Autodesk Inventor part; units mm, degrees
(part 4 of 4)
sketch "Sketch7" plane through (0, 0, 2) normal (0, 0, 1) x (1, 0, 0)
  arc A0 (20.5, -320) -> (16, -320) centre (18.25, -320) ccw projected
  line L0 (20.5, -320) -> (20.5, -360) projected
  arc A1 (16, -360) -> (20.5, -360) centre (18.25, -360) ccw projected
  line L1 (16, -360) -> (16, -320) projected
  arc A2 (12.5, -320) -> (8, -320) centre (10.25, -320) ccw projected
  line L2 (12.5, -320) -> (12.5, -360) projected
  arc A3 (8, -360) -> (12.5, -360) centre (10.25, -360) ccw projected
  line L3 (8, -360) -> (8, -320) projected
  arc A4 (0, -360) -> (4.5, -360) centre (2.25, -360) ccw projected
  line L4 (0, -360) -> (0, -320) projected
  arc A5 (4.5, -320) -> (0, -320) centre (2.25, -320) ccw projected
  line L5 (4.5, -320) -> (4.5, -360) projected
  line L6 (283.7872, -294.4284) -> (283.7872, -329.9768) projected
  line L7 (283.7872, -329.9768) -> (273.4247, -329.9768) projected
  line L8 (273.4247, -329.9768) -> (267.105, -323.7035) projected
  line L9 (267.105, -323.7035) -> (267.105, -286.25) projected
  line L10 (267.105, -286.25) -> (273.4247, -279.9768) projected
  line L11 (273.4247, -279.9768) -> (299.54, -279.9768) projected
  line L12 (299.54, -279.9768) -> (299.54, -294.4284) projected
  line L13 (299.54, -294.4284) -> (283.7872, -294.4284) projected
  line L14 (242.9879, -315.1998) -> (242.9879, -330.0232) projected
  line L15 (242.9879, -330.0232) -> (227.2351, -330.0232) projected
  line L16 (227.2351, -330.0232) -> (210.553, -313.3411) projected
  line L17 (210.553, -313.3411) -> (210.553, -279.9768) projected
  line L18 (210.553, -279.9768) -> (227.2351, -279.9768) projected
  line L19 (227.2351, -279.9768) -> (227.2351, -315.1998) projected
  line L20 (227.2351, -315.1998) -> (242.9879, -315.1998) projected
  line L21 (206.2779, -316.1756) -> (206.2779, -329.9768) projected
  line L22 (206.2779, -329.9768) -> (173.8429, -329.9768) projected
  line L23 (173.8429, -329.9768) -> (173.8429, -316.1756) projected
  line L24 (173.8429, -316.1756) -> (206.2779, -316.1756) projected
  line L25 (170.3113, -279.9768) -> (170.3113, -329.9768) projected
  line L26 (170.3113, -329.9768) -> (159.9954, -329.9768) projected
  line L27 (159.9954, -329.9768) -> (153.7221, -323.7035) projected
  line L28 (153.7221, -323.7035) -> (153.7221, -286.25) projected
  line L29 (153.7221, -286.25) -> (159.9954, -279.9768) projected
  line L30 (159.9954, -279.9768) -> (170.3113, -279.9768) projected
  line L31 (129.3262, -316.1292) -> (129.3262, -329.9303) projected
  line L32 (129.3262, -329.9303) -> (104.7444, -329.9303) projected
  line L33 (104.7444, -329.9303) -> (96.8913, -322.0771) projected
  line L34 (96.8913, -322.0771) -> (96.8913, -294.289) projected
  line L35 (96.8913, -294.289) -> (113.5734, -294.289) projected
  line L36 (113.5734, -294.289) -> (113.5734, -316.1292) projected
  line L37 (113.5734, -316.1292) -> (129.3262, -316.1292) projected
  line L38 (56.789, -329.9768) -> (46.6125, -329.9768) projected
  line L39 (46.6125, -329.9768) -> (40.3392, -323.7035) projected
  line L40 (40.3392, -323.7035) -> (40.3392, -279.9768) projected
  line L41 (40.3392, -279.9768) -> (56.789, -279.9768) projected
  line L42 (56.789, -279.9768) -> (56.789, -329.9768) projected
  line L43 (92.5697, -329.9768) -> (60.3206, -329.9768) projected
  line L44 (60.3206, -329.9768) -> (60.3206, -316.1756) projected
  line L45 (60.3206, -316.1756) -> (92.5697, -316.1756) projected
  line L46 (92.5697, -316.1756) -> (92.5697, -329.9768) projected
  line L47 (149.447, -294.289) -> (149.447, -329.9303) projected
  line L48 (149.447, -329.9303) -> (132.7649, -329.9303) projected
  line L49 (132.7649, -329.9303) -> (132.7649, -294.289) projected
  line L50 (132.7649, -294.289) -> (149.447, -294.289) projected
  line L51 (206.2779, -279.9768) -> (206.2779, -294.4284) projected
  line L52 (206.2779, -294.4284) -> (173.8429, -294.4284) projected
  line L53 (173.8429, -294.4284) -> (173.8429, -279.9768) projected
  line L54 (173.8429, -279.9768) -> (206.2779, -279.9768) projected
  line L55 (206.2779, -297.96) -> (206.2779, -308.973) projected
  line L56 (206.2779, -308.973) -> (173.8429, -308.973) projected
  line L57 (173.8429, -308.973) -> (173.8429, -297.96) projected
  line L58 (173.8429, -297.96) -> (206.2779, -297.96) projected
  line L59 (262.8299, -313.3411) -> (246.4266, -329.9768) projected
  line L60 (246.4266, -329.9768) -> (246.4266, -279.9768) projected
  line L61 (246.4266, -279.9768) -> (262.8299, -279.9768) projected
  line L62 (262.8299, -279.9768) -> (262.8299, -313.3411) projected
  line L63 (319.6608, -286.25) -> (319.6608, -323.7035) projected
  line L64 (319.6608, -323.7035) -> (313.3411, -329.9768) projected
  line L65 (313.3411, -329.9768) -> (287.1794, -329.9768) projected
  line L66 (287.1794, -329.9768) -> (287.1794, -316.1756) projected
  line L67 (287.1794, -316.1756) -> (302.9786, -316.1756) projected
  line L68 (302.9786, -316.1756) -> (302.9786, -279.9768) projected
  line L69 (302.9786, -279.9768) -> (313.3411, -279.9768) projected
  line L70 (313.3411, -279.9768) -> (319.6608, -286.25) projected
  line L71 (31.2247, -413) -> (28.338, -408) projected
  line L72 (28.338, -408) -> (31.2247, -403) projected
  line L73 (31.2247, -403) -> (36.9983, -403) projected
  line L74 (36.9983, -403) -> (39.885, -408) projected
  line L75 (39.885, -408) -> (36.9983, -413) projected
  line L76 (36.9983, -413) -> (31.2247, -413) projected
  line L77 (49.9886, -440.5) -> (52.8754, -445.5) projected
  line L78 (52.8754, -445.5) -> (49.9886, -450.5) projected
  line L79 (49.9886, -450.5) -> (44.2151, -450.5) projected
  line L80 (44.2151, -450.5) -> (41.3284, -445.5) projected
  line L81 (41.3284, -445.5) -> (44.2151, -440.5) projected
  line L82 (44.2151, -440.5) -> (49.9886, -440.5) projected
  line L83 (57.2247, -418) -> (62.9983, -418) projected
  line L84 (62.9983, -418) -> (65.885, -423) projected
  line L85 (65.885, -423) -> (62.9983, -428) projected
  line L86 (62.9983, -428) -> (57.2247, -428) projected
  line L87 (57.2247, -428) -> (54.338, -423) projected
  line L88 (54.338, -423) -> (57.2247, -418) projected
  line L89 (78.8754, -430.5) -> (75.9886, -435.5) projected
  line L90 (75.9886, -435.5) -> (70.2151, -435.5) projected
  line L91 (70.2151, -435.5) -> (67.3284, -430.5) projected
  line L92 (67.3284, -430.5) -> (70.2151, -425.5) projected
  line L93 (70.2151, -425.5) -> (75.9886, -425.5) projected
  line L94 (75.9886, -425.5) -> (78.8754, -430.5) projected
  line L95 (80.338, -438) -> (83.2247, -433) projected
  line L96 (83.2247, -433) -> (88.9983, -433) projected
  line L97 (88.9983, -433) -> (91.885, -438) projected
  line L98 (91.885, -438) -> (88.9983, -443) projected
  line L99 (88.9983, -443) -> (83.2247, -443) projected
  line L100 (83.2247, -443) -> (80.338, -438) projected
  line L101 (101.9886, -410.5) -> (104.8754, -415.5) projected
  line L102 (104.8754, -415.5) -> (101.9886, -420.5) projected
  line L103 (101.9886, -420.5) -> (96.2151, -420.5) projected
  line L104 (96.2151, -420.5) -> (93.3284, -415.5) projected
  line L105 (93.3284, -415.5) -> (96.2151, -410.5) projected
  line L106 (96.2151, -410.5) -> (101.9886, -410.5) projected
  line L107 (109.2247, -448) -> (114.9983, -448) projected
  line L108 (114.9983, -448) -> (117.885, -453) projected
  line L109 (117.885, -453) -> (114.9983, -458) projected
  line L110 (114.9983, -458) -> (109.2247, -458) projected
  line L111 (109.2247, -458) -> (106.338, -453) projected
  line L112 (106.338, -453) -> (109.2247, -448) projected
  line L113 (135.2247, -413) -> (132.338, -408) projected
  line L114 (132.338, -408) -> (135.2247, -403) projected
  line L115 (135.2247, -403) -> (140.9983, -403) projected
  line L116 (140.9983, -403) -> (143.885, -408) projected
  line L117 (143.885, -408) -> (140.9983, -413) projected
  line L118 (140.9983, -413) -> (135.2247, -413) projected
  line L119 (153.9886, -440.5) -> (156.8754, -445.5) projected
  line L120 (156.8754, -445.5) -> (153.9886, -450.5) projected
  line L121 (153.9886, -450.5) -> (148.2151, -450.5) projected
  line L122 (148.2151, -450.5) -> (145.3284, -445.5) projected
  line L123 (145.3284, -445.5) -> (148.2151, -440.5) projected
  line L124 (148.2151, -440.5) -> (153.9886, -440.5) projected
  line L125 (153.9886, -410.5) -> (156.8754, -415.5) projected
  line L126 (156.8754, -415.5) -> (153.9886, -420.5) projected
  line L127 (153.9886, -420.5) -> (148.2151, -420.5) projected
  line L128 (148.2151, -420.5) -> (145.3284, -415.5) projected
  line L129 (145.3284, -415.5) -> (148.2151, -410.5) projected
  line L130 (148.2151, -410.5) -> (153.9886, -410.5) projected
  line L131 (182.8754, -430.5) -> (179.9886, -435.5) projected
  line L132 (179.9886, -435.5) -> (174.2151, -435.5) projected
  line L133 (174.2151, -435.5) -> (171.3284, -430.5) projected
  line L134 (171.3284, -430.5) -> (174.2151, -425.5) projected
  line L135 (174.2151, -425.5) -> (179.9886, -425.5) projected
  line L136 (179.9886, -425.5) -> (182.8754, -430.5) projected
  line L137 (184.338, -438) -> (187.2247, -433) projected
  line L138 (187.2247, -433) -> (192.9983, -433) projected
  line L139 (192.9983, -433) -> (195.885, -438) projected
  line L140 (195.885, -438) -> (192.9983, -443) projected
  line L141 (192.9983, -443) -> (187.2247, -443) projected
  line L142 (187.2247, -443) -> (184.338, -438) projected
  line L143 (205.9886, -410.5) -> (208.8754, -415.5) projected
  line L144 (208.8754, -415.5) -> (205.9886, -420.5) projected
  line L145 (205.9886, -420.5) -> (200.2151, -420.5) projected
  line L146 (200.2151, -420.5) -> (197.3284, -415.5) projected
  line L147 (197.3284, -415.5) -> (200.2151, -410.5) projected
  line L148 (200.2151, -410.5) -> (205.9886, -410.5) projected
  line L149 (213.2247, -448) -> (218.9983, -448) projected
  line L150 (218.9983, -448) -> (221.885, -453) projected
  line L151 (221.885, -453) -> (218.9983, -458) projected
  line L152 (218.9983, -458) -> (213.2247, -458) projected
  line L153 (213.2247, -458) -> (210.338, -453) projected
  line L154 (210.338, -453) -> (213.2247, -448) projected
  line L155 (239.2247, -413) -> (236.338, -408) projected
  line L156 (236.338, -408) -> (239.2247, -403) projected
  line L157 (239.2247, -403) -> (244.9983, -403) projected
  line L158 (244.9983, -403) -> (247.885, -408) projected
  line L159 (247.885, -408) -> (244.9983, -413) projected
  line L160 (244.9983, -413) -> (239.2247, -413) projected
  line L161 (257.9886, -440.5) -> (260.8754, -445.5) projected
  line L162 (260.8754, -445.5) -> (257.9886, -450.5) projected
  line L163 (257.9886, -450.5) -> (252.2151, -450.5) projected
  line L164 (252.2151, -450.5) -> (249.3284, -445.5) projected
  line L165 (249.3284, -445.5) -> (252.2151, -440.5) projected
  line L166 (252.2151, -440.5) -> (257.9886, -440.5) projected
  line L167 (265.2247, -418) -> (270.9983, -418) projected
  line L168 (270.9983, -418) -> (273.885, -423) projected
  line L169 (273.885, -423) -> (270.9983, -428) projected
  line L170 (270.9983, -428) -> (265.2247, -428) projected
  line L171 (265.2247, -428) -> (262.338, -423) projected
  line L172 (262.338, -423) -> (265.2247, -418) projected
  line L173 (291.2247, -448) -> (296.9983, -448) projected
  line L174 (296.9983, -448) -> (299.885, -453) projected
  line L175 (299.885, -453) -> (296.9983, -458) projected
  line L176 (296.9983, -458) -> (291.2247, -458) projected
  line L177 (291.2247, -458) -> (288.338, -453) projected
  line L178 (288.338, -453) -> (291.2247, -448) projected
  line L179 (343.2247, -448) -> (348.9983, -448) projected
  line L180 (348.9983, -448) -> (351.885, -453) projected
  line L181 (351.885, -453) -> (348.9983, -458) projected
  line L182 (348.9983, -458) -> (343.2247, -458) projected
  line L183 (343.2247, -458) -> (340.338, -453) projected
  line L184 (340.338, -453) -> (343.2247, -448) projected
  line L185 (335.9886, -410.5) -> (338.8754, -415.5) projected
  line L186 (338.8754, -415.5) -> (335.9886, -420.5) projected
  line L187 (335.9886, -420.5) -> (330.2151, -420.5) projected
  line L188 (330.2151, -420.5) -> (327.3284, -415.5) projected
  line L189 (327.3284, -415.5) -> (330.2151, -410.5) projected
  line L190 (330.2151, -410.5) -> (335.9886, -410.5) projected
  line L191 (286.8754, -430.5) -> (283.9886, -435.5) projected
  line L192 (283.9886, -435.5) -> (278.2151, -435.5) projected
  line L193 (278.2151, -435.5) -> (275.3284, -430.5) projected
  line L194 (275.3284, -430.5) -> (278.2151, -425.5) projected
  line L195 (278.2151, -425.5) -> (283.9886, -425.5) projected
  line L196 (283.9886, -425.5) -> (286.8754, -430.5) projected
  line L197 (309.9886, -410.5) -> (312.8754, -415.5) projected
  line L198 (312.8754, -415.5) -> (309.9886, -420.5) projected
  line L199 (309.9886, -420.5) -> (304.2151, -420.5) projected
  line L200 (304.2151, -420.5) -> (301.3284, -415.5) projected
  line L201 (301.3284, -415.5) -> (304.2151, -410.5) projected
  line L202 (304.2151, -410.5) -> (309.9886, -410.5) projected
  line L203 (5.2247, -433) -> (10.9983, -433) projected
  line L204 (10.9983, -433) -> (13.885, -438) projected
  line L205 (13.885, -438) -> (10.9983, -443) projected
  line L206 (10.9983, -443) -> (5.2247, -443) projected
  line L207 (5.2247, -443) -> (2.338, -438) projected
  line L208 (2.338, -438) -> (5.2247, -433) projected
  line L209 (23.9886, -440.5) -> (26.8754, -445.5) projected
  line L210 (26.8754, -445.5) -> (23.9886, -450.5) projected
  line L211 (23.9886, -450.5) -> (18.2151, -450.5) projected
  line L212 (18.2151, -450.5) -> (15.3284, -445.5) projected
  line L213 (15.3284, -445.5) -> (18.2151, -440.5) projected
  line L214 (18.2151, -440.5) -> (23.9886, -440.5) projected
  line L215 (10.9983, -428) -> (5.2247, -428) projected
  line L216 (5.2247, -428) -> (2.338, -423) projected
  line L217 (2.338, -423) -> (5.2247, -418) projected
  line L218 (5.2247, -418) -> (10.9983, -418) projected
  line L219 (10.9983, -418) -> (13.885, -423) projected
  line L220 (13.885, -423) -> (10.9983, -428) projected
  line L221 (317.2247, -418) -> (322.9983, -418) projected
  line L222 (322.9983, -418) -> (325.885, -423) projected
  line L223 (325.885, -423) -> (322.9983, -428) projected
  line L224 (322.9983, -428) -> (317.2247, -428) projected
  line L225 (317.2247, -428) -> (314.338, -423) projected
  line L226 (314.338, -423) -> (317.2247, -418) projected
  line L227 (291.2247, -418) -> (296.9983, -418) projected
  line L228 (296.9983, -418) -> (299.885, -423) projected
  line L229 (299.885, -423) -> (296.9983, -428) projected
  line L230 (296.9983, -428) -> (291.2247, -428) projected
  line L231 (291.2247, -428) -> (288.338, -423) projected
  line L232 (288.338, -423) -> (291.2247, -418) projected
  line L233 (317.2247, -413) -> (314.338, -408) projected
  line L234 (314.338, -408) -> (317.2247, -403) projected
  line L235 (317.2247, -403) -> (322.9983, -403) projected
  line L236 (322.9983, -403) -> (325.885, -408) projected
  line L237 (325.885, -408) -> (322.9983, -413) projected
  line L238 (322.9983, -413) -> (317.2247, -413) projected
  line L239 (340.338, -438) -> (343.2247, -433) projected
  line L240 (343.2247, -433) -> (348.9983, -433) projected
  line L241 (348.9983, -433) -> (351.885, -438) projected
  line L242 (351.885, -438) -> (348.9983, -443) projected
  line L243 (348.9983, -443) -> (343.2247, -443) projected
  line L244 (343.2247, -443) -> (340.338, -438) projected
  line L245 (309.9886, -440.5) -> (312.8754, -445.5) projected
  line L246 (312.8754, -445.5) -> (309.9886, -450.5) projected
  line L247 (309.9886, -450.5) -> (304.2151, -450.5) projected
  line L248 (304.2151, -450.5) -> (301.3284, -445.5) projected
  line L249 (301.3284, -445.5) -> (304.2151, -440.5) projected
  line L250 (304.2151, -440.5) -> (309.9886, -440.5) projected
  line L251 (262.338, -438) -> (265.2247, -433) projected
  line L252 (265.2247, -433) -> (270.9983, -433) projected
  line L253 (270.9983, -433) -> (273.885, -438) projected
  line L254 (273.885, -438) -> (270.9983, -443) projected
  line L255 (270.9983, -443) -> (265.2247, -443) projected
  line L256 (265.2247, -443) -> (262.338, -438) projected
  line L257 (260.8754, -430.5) -> (257.9886, -435.5) projected
  line L258 (257.9886, -435.5) -> (252.2151, -435.5) projected
  line L259 (252.2151, -435.5) -> (249.3284, -430.5) projected
  line L260 (249.3284, -430.5) -> (252.2151, -425.5) projected
  line L261 (252.2151, -425.5) -> (257.9886, -425.5) projected
  line L262 (257.9886, -425.5) -> (260.8754, -430.5) projected
  line L263 (239.2247, -418) -> (244.9983, -418) projected
  line L264 (244.9983, -418) -> (247.885, -423) projected
  line L265 (247.885, -423) -> (244.9983, -428) projected
  line L266 (244.9983, -428) -> (239.2247, -428) projected
  line L267 (239.2247, -428) -> (236.338, -423) projected
  line L268 (236.338, -423) -> (239.2247, -418) projected
  line L269 (231.9886, -440.5) -> (234.8754, -445.5) projected
  line L270 (234.8754, -445.5) -> (231.9886, -450.5) projected
  line L271 (231.9886, -450.5) -> (226.2151, -450.5) projected
  line L272 (226.2151, -450.5) -> (223.3284, -445.5) projected
  line L273 (223.3284, -445.5) -> (226.2151, -440.5) projected
  line L274 (226.2151, -440.5) -> (231.9886, -440.5) projected
  line L275 (213.2247, -413) -> (210.338, -408) projected
  line L276 (210.338, -408) -> (213.2247, -403) projected
  line L277 (213.2247, -403) -> (218.9983, -403) projected
  line L278 (218.9983, -403) -> (221.885, -408) projected
  line L279 (221.885, -408) -> (218.9983, -413) projected
  line L280 (218.9983, -413) -> (213.2247, -413) projected
  line L281 (187.2247, -448) -> (192.9983, -448) projected
  line L282 (192.9983, -448) -> (195.885, -453) projected
  line L283 (195.885, -453) -> (192.9983, -458) projected
  line L284 (192.9983, -458) -> (187.2247, -458) projected
  line L285 (187.2247, -458) -> (184.338, -453) projected
  line L286 (184.338, -453) -> (187.2247, -448) projected
  line L287 (179.9886, -410.5) -> (182.8754, -415.5) projected
  line L288 (182.8754, -415.5) -> (179.9886, -420.5) projected
  line L289 (179.9886, -420.5) -> (174.2151, -420.5) projected
  line L290 (174.2151, -420.5) -> (171.3284, -415.5) projected
  line L291 (171.3284, -415.5) -> (174.2151, -410.5) projected
  line L292 (174.2151, -410.5) -> (179.9886, -410.5) projected
  line L293 (161.2247, -413) -> (158.338, -408) projected
  line L294 (158.338, -408) -> (161.2247, -403) projected
  line L295 (161.2247, -403) -> (166.9983, -403) projected
  line L296 (166.9983, -403) -> (169.885, -408) projected
  line L297 (169.885, -408) -> (166.9983, -413) projected
  line L298 (166.9983, -413) -> (161.2247, -413) projected
  line L299 (161.2247, -448) -> (166.9983, -448) projected
  line L300 (166.9983, -448) -> (169.885, -453) projected
  line L301 (169.885, -453) -> (166.9983, -458) projected
  line L302 (166.9983, -458) -> (161.2247, -458) projected
  line L303 (161.2247, -458) -> (158.338, -453) projected
  line L304 (158.338, -453) -> (161.2247, -448) projected
  line L305 (135.2247, -418) -> (140.9983, -418) projected
  line L306 (140.9983, -418) -> (143.885, -423) projected
  line L307 (143.885, -423) -> (140.9983, -428) projected
  line L308 (140.9983, -428) -> (135.2247, -428) projected
  line L309 (135.2247, -428) -> (132.338, -423) projected
  line L310 (132.338, -423) -> (135.2247, -418) projected
  line L311 (127.9886, -440.5) -> (130.8754, -445.5) projected
  line L312 (130.8754, -445.5) -> (127.9886, -450.5) projected
  line L313 (127.9886, -450.5) -> (122.2151, -450.5) projected
  line L314 (122.2151, -450.5) -> (119.3284, -445.5) projected
  line L315 (119.3284, -445.5) -> (122.2151, -440.5) projected
  line L316 (122.2151, -440.5) -> (127.9886, -440.5) projected
  line L317 (109.2247, -413) -> (106.338, -408) projected
  line L318 (106.338, -408) -> (109.2247, -403) projected
  line L319 (109.2247, -403) -> (114.9983, -403) projected
  line L320 (114.9983, -403) -> (117.885, -408) projected
  line L321 (117.885, -408) -> (114.9983, -413) projected
  line L322 (114.9983, -413) -> (109.2247, -413) projected
  line L323 (83.2247, -448) -> (88.9983, -448) projected
  line L324 (88.9983, -448) -> (91.885, -453) projected
  line L325 (91.885, -453) -> (88.9983, -458) projected
  line L326 (88.9983, -458) -> (83.2247, -458) projected
  line L327 (83.2247, -458) -> (80.338, -453) projected
  line L328 (80.338, -453) -> (83.2247, -448) projected
  line L329 (75.9886, -410.5) -> (78.8754, -415.5) projected
  line L330 (78.8754, -415.5) -> (75.9886, -420.5) projected
  line L331 (75.9886, -420.5) -> (70.2151, -420.5) projected
  line L332 (70.2151, -420.5) -> (67.3284, -415.5) projected
  line L333 (67.3284, -415.5) -> (70.2151, -410.5) projected
  line L334 (70.2151, -410.5) -> (75.9886, -410.5) projected
  line L335 (54.338, -438) -> (57.2247, -433) projected
  line L336 (57.2247, -433) -> (62.9983, -433) projected
  line L337 (62.9983, -433) -> (65.885, -438) projected
  line L338 (65.885, -438) -> (62.9983, -443) projected
  line L339 (62.9983, -443) -> (57.2247, -443) projected
  line L340 (57.2247, -443) -> (54.338, -438) projected
  line L341 (52.8754, -430.5) -> (49.9886, -435.5) projected
  line L342 (49.9886, -435.5) -> (44.2151, -435.5) projected
  line L343 (44.2151, -435.5) -> (41.3284, -430.5) projected
  line L344 (41.3284, -430.5) -> (44.2151, -425.5) projected
  line L345 (44.2151, -425.5) -> (49.9886, -425.5) projected
  line L346 (49.9886, -425.5) -> (52.8754, -430.5) projected
  line L347 (31.2247, -418) -> (36.9983, -418) projected
  line L348 (36.9983, -418) -> (39.885, -423) projected
  line L349 (39.885, -423) -> (36.9983, -428) projected
  line L350 (36.9983, -428) -> (31.2247, -428) projected
  line L351 (31.2247, -428) -> (28.338, -423) projected
  line L352 (28.338, -423) -> (31.2247, -418) projected
  line L353 (23.9886, -420.5) -> (18.2151, -420.5) projected
  line L354 (18.2151, -420.5) -> (15.3284, -415.5) projected
  line L355 (15.3284, -415.5) -> (18.2151, -410.5) projected
  line L356 (18.2151, -410.5) -> (23.9886, -410.5) projected
  line L357 (23.9886, -410.5) -> (26.8754, -415.5) projected
  line L358 (26.8754, -415.5) -> (23.9886, -420.5) projected
  line L359 (31.2247, -448) -> (36.9983, -448) projected
  line L360 (36.9983, -448) -> (39.885, -453) projected
  line L361 (39.885, -453) -> (36.9983, -458) projected
  line L362 (36.9983, -458) -> (31.2247, -458) projected
  line L363 (31.2247, -458) -> (28.338, -453) projected
  line L364 (28.338, -453) -> (31.2247, -448) projected
  line L365 (57.2247, -413) -> (54.338, -408) projected
  line L366 (54.338, -408) -> (57.2247, -403) projected
  line L367 (57.2247, -403) -> (62.9983, -403) projected
  line L368 (62.9983, -403) -> (65.885, -408) projected
  line L369 (65.885, -408) -> (62.9983, -413) projected
  line L370 (62.9983, -413) -> (57.2247, -413) projected
  line L371 (75.9886, -440.5) -> (78.8754, -445.5) projected
  line L372 (78.8754, -445.5) -> (75.9886, -450.5) projected
  line L373 (75.9886, -450.5) -> (70.2151, -450.5) projected
  line L374 (70.2151, -450.5) -> (67.3284, -445.5) projected
  line L375 (67.3284, -445.5) -> (70.2151, -440.5) projected
  line L376 (70.2151, -440.5) -> (75.9886, -440.5) projected
  line L377 (83.2247, -418) -> (88.9983, -418) projected
  line L378 (88.9983, -418) -> (91.885, -423) projected
  line L379 (91.885, -423) -> (88.9983, -428) projected
  line L380 (88.9983, -428) -> (83.2247, -428) projected
  line L381 (83.2247, -428) -> (80.338, -423) projected
  line L382 (80.338, -423) -> (83.2247, -418) projected
  line L383 (104.8754, -430.5) -> (101.9886, -435.5) projected
  line L384 (101.9886, -435.5) -> (96.2151, -435.5) projected
  line L385 (96.2151, -435.5) -> (93.3284, -430.5) projected
  line L386 (93.3284, -430.5) -> (96.2151, -425.5) projected
  line L387 (96.2151, -425.5) -> (101.9886, -425.5) projected
  line L388 (101.9886, -425.5) -> (104.8754, -430.5) projected
  line L389 (106.338, -438) -> (109.2247, -433) projected
  line L390 (109.2247, -433) -> (114.9983, -433) projected
  line L391 (114.9983, -433) -> (117.885, -438) projected
  line L392 (117.885, -438) -> (114.9983, -443) projected
  line L393 (114.9983, -443) -> (109.2247, -443) projected
  line L394 (109.2247, -443) -> (106.338, -438) projected
  line L395 (127.9886, -410.5) -> (130.8754, -415.5) projected
  line L396 (130.8754, -415.5) -> (127.9886, -420.5) projected
  line L397 (127.9886, -420.5) -> (122.2151, -420.5) projected
  line L398 (122.2151, -420.5) -> (119.3284, -415.5) projected
  line L399 (119.3284, -415.5) -> (122.2151, -410.5) projected
  line L400 (122.2151, -410.5) -> (127.9886, -410.5) projected
  line L401 (135.2247, -448) -> (140.9983, -448) projected
  line L402 (140.9983, -448) -> (143.885, -453) projected
  line L403 (143.885, -453) -> (140.9983, -458) projected
  line L404 (140.9983, -458) -> (135.2247, -458) projected
  line L405 (135.2247, -458) -> (132.338, -453) projected
  line L406 (132.338, -453) -> (135.2247, -448) projected
  line L407 (156.8754, -430.5) -> (153.9886, -435.5) projected
  line L408 (153.9886, -435.5) -> (148.2151, -435.5) projected
  line L409 (148.2151, -435.5) -> (145.3284, -430.5) projected
  line L410 (145.3284, -430.5) -> (148.2151, -425.5) projected
  line L411 (148.2151, -425.5) -> (153.9886, -425.5) projected
  line L412 (153.9886, -425.5) -> (156.8754, -430.5) projected
  line L413 (179.9886, -440.5) -> (182.8754, -445.5) projected
  line L414 (182.8754, -445.5) -> (179.9886, -450.5) projected
  line L415 (179.9886, -450.5) -> (174.2151, -450.5) projected
  line L416 (174.2151, -450.5) -> (171.3284, -445.5) projected
  line L417 (171.3284, -445.5) -> (174.2151, -440.5) projected
  line L418 (174.2151, -440.5) -> (179.9886, -440.5) projected
  line L419 (187.2247, -418) -> (192.9983, -418) projected
  line L420 (192.9983, -418) -> (195.885, -423) projected
  line L421 (195.885, -423) -> (192.9983, -428) projected
  line L422 (192.9983, -428) -> (187.2247, -428) projected
  line L423 (187.2247, -428) -> (184.338, -423) projected
  line L424 (184.338, -423) -> (187.2247, -418) projected
  line L425 (208.8754, -430.5) -> (205.9886, -435.5) projected
  line L426 (205.9886, -435.5) -> (200.2151, -435.5) projected
  line L427 (200.2151, -435.5) -> (197.3284, -430.5) projected
  line L428 (197.3284, -430.5) -> (200.2151, -425.5) projected
  line L429 (200.2151, -425.5) -> (205.9886, -425.5) projected
  line L430 (205.9886, -425.5) -> (208.8754, -430.5) projected
  line L431 (210.338, -438) -> (213.2247, -433) projected
  line L432 (213.2247, -433) -> (218.9983, -433) projected
  line L433 (218.9983, -433) -> (221.885, -438) projected
  line L434 (221.885, -438) -> (218.9983, -443) projected
  line L435 (218.9983, -443) -> (213.2247, -443) projected
  line L436 (213.2247, -443) -> (210.338, -438) projected
  line L437 (231.9886, -410.5) -> (234.8754, -415.5) projected
  line L438 (234.8754, -415.5) -> (231.9886, -420.5) projected
  line L439 (231.9886, -420.5) -> (226.2151, -420.5) projected
  line L440 (226.2151, -420.5) -> (223.3284, -415.5) projected
  line L441 (223.3284, -415.5) -> (226.2151, -410.5) projected
  line L442 (226.2151, -410.5) -> (231.9886, -410.5) projected
  line L443 (239.2247, -448) -> (244.9983, -448) projected
  line L444 (244.9983, -448) -> (247.885, -453) projected
  line L445 (247.885, -453) -> (244.9983, -458) projected
  line L446 (244.9983, -458) -> (239.2247, -458) projected
  line L447 (239.2247, -458) -> (236.338, -453) projected
  line L448 (236.338, -453) -> (239.2247, -448) projected
  line L449 (265.2247, -413) -> (262.338, -408) projected
  line L450 (262.338, -408) -> (265.2247, -403) projected
  line L451 (265.2247, -403) -> (270.9983, -403) projected
  line L452 (270.9983, -403) -> (273.885, -408) projected
  line L453 (273.885, -408) -> (270.9983, -413) projected
  line L454 (270.9983, -413) -> (265.2247, -413) projected
  line L455 (283.9886, -440.5) -> (286.8754, -445.5) projected
  line L456 (286.8754, -445.5) -> (283.9886, -450.5) projected
  line L457 (283.9886, -450.5) -> (278.2151, -450.5) projected
  line L458 (278.2151, -450.5) -> (275.3284, -445.5) projected
  line L459 (275.3284, -445.5) -> (278.2151, -440.5) projected
  line L460 (278.2151, -440.5) -> (283.9886, -440.5) projected
  line L461 (335.9886, -440.5) -> (338.8754, -445.5) projected
  line L462 (338.8754, -445.5) -> (335.9886, -450.5) projected
  line L463 (335.9886, -450.5) -> (330.2151, -450.5) projected
  line L464 (330.2151, -450.5) -> (327.3284, -445.5) projected
  line L465 (327.3284, -445.5) -> (330.2151, -440.5) projected
  line L466 (330.2151, -440.5) -> (335.9886, -440.5) projected
  line L467 (343.2247, -413) -> (340.338, -408) projected
  line L468 (340.338, -408) -> (343.2247, -403) projected
  line L469 (343.2247, -403) -> (348.9983, -403) projected
  line L470 (348.9983, -403) -> (351.885, -408) projected
  line L471 (351.885, -408) -> (348.9983, -413) projected
  line L472 (348.9983, -413) -> (343.2247, -413) projected
  line L473 (283.9886, -410.5) -> (286.8754, -415.5) projected
  line L474 (286.8754, -415.5) -> (283.9886, -420.5) projected
  line L475 (283.9886, -420.5) -> (278.2151, -420.5) projected
  line L476 (278.2151, -420.5) -> (275.3284, -415.5) projected
  line L477 (275.3284, -415.5) -> (278.2151, -410.5) projected
  line L478 (278.2151, -410.5) -> (283.9886, -410.5) projected
  line L479 (312.8754, -430.5) -> (309.9886, -435.5) projected
  line L480 (309.9886, -435.5) -> (304.2151, -435.5) projected
  line L481 (304.2151, -435.5) -> (301.3284, -430.5) projected
  line L482 (301.3284, -430.5) -> (304.2151, -425.5) projected
  line L483 (304.2151, -425.5) -> (309.9886, -425.5) projected
  line L484 (309.9886, -425.5) -> (312.8754, -430.5) projected
  line L485 (338.8754, -430.5) -> (335.9886, -435.5) projected
  line L486 (335.9886, -435.5) -> (330.2151, -435.5) projected
  line L487 (330.2151, -435.5) -> (327.3284, -430.5) projected
  line L488 (327.3284, -430.5) -> (330.2151, -425.5) projected
  line L489 (330.2151, -425.5) -> (335.9886, -425.5) projected
  line L490 (335.9886, -425.5) -> (338.8754, -430.5) projected
  line L491 (23.9886, -435.5) -> (18.2151, -435.5) projected
  line L492 (18.2151, -435.5) -> (15.3284, -430.5) projected
  line L493 (15.3284, -430.5) -> (18.2151, -425.5) projected
  line L494 (18.2151, -425.5) -> (23.9886, -425.5) projected
  line L495 (23.9886, -425.5) -> (26.8754, -430.5) projected
  line L496 (26.8754, -430.5) -> (23.9886, -435.5) projected
  line L497 (5.2247, -448) -> (10.9983, -448) projected
  line L498 (10.9983, -448) -> (13.885, -453) projected
  line L499 (13.885, -453) -> (10.9983, -458) projected
  line L500 (10.9983, -458) -> (5.2247, -458) projected
  line L501 (5.2247, -458) -> (2.338, -453) projected
  line L502 (2.338, -453) -> (5.2247, -448) projected
  line L503 (314.338, -438) -> (317.2247, -433) projected
  line L504 (317.2247, -433) -> (322.9983, -433) projected
  line L505 (322.9983, -433) -> (325.885, -438) projected
  line L506 (325.885, -438) -> (322.9983, -443) projected
  line L507 (322.9983, -443) -> (317.2247, -443) projected
  line L508 (317.2247, -443) -> (314.338, -438) projected
  line L509 (288.338, -438) -> (291.2247, -433) projected
  line L510 (291.2247, -433) -> (296.9983, -433) projected
  line L511 (296.9983, -433) -> (299.885, -438) projected
  line L512 (299.885, -438) -> (296.9983, -443) projected
  line L513 (296.9983, -443) -> (291.2247, -443) projected
  line L514 (291.2247, -443) -> (288.338, -438) projected
  line L515 (291.2247, -413) -> (288.338, -408) projected
  line L516 (288.338, -408) -> (291.2247, -403) projected
  line L517 (291.2247, -403) -> (296.9983, -403) projected
  line L518 (296.9983, -403) -> (299.885, -408) projected
  line L519 (299.885, -408) -> (296.9983, -413) projected
  line L520 (296.9983, -413) -> (291.2247, -413) projected
  line L521 (343.2247, -418) -> (348.9983, -418) projected
  line L522 (348.9983, -418) -> (351.885, -423) projected
  line L523 (351.885, -423) -> (348.9983, -428) projected
  line L524 (348.9983, -428) -> (343.2247, -428) projected
  line L525 (343.2247, -428) -> (340.338, -423) projected
  line L526 (340.338, -423) -> (343.2247, -418) projected
  line L527 (317.2247, -448) -> (322.9983, -448) projected
  line L528 (322.9983, -448) -> (325.885, -453) projected
  line L529 (325.885, -453) -> (322.9983, -458) projected
  line L530 (322.9983, -458) -> (317.2247, -458) projected
  line L531 (317.2247, -458) -> (314.338, -453) projected
  line L532 (314.338, -453) -> (317.2247, -448) projected
  line L533 (265.2247, -448) -> (270.9983, -448) projected
  line L534 (270.9983, -448) -> (273.885, -453) projected
  line L535 (273.885, -453) -> (270.9983, -458) projected
  line L536 (270.9983, -458) -> (265.2247, -458) projected
  line L537 (265.2247, -458) -> (262.338, -453) projected
  line L538 (262.338, -453) -> (265.2247, -448) projected
  line L539 (257.9886, -410.5) -> (260.8754, -415.5) projected
  line L540 (260.8754, -415.5) -> (257.9886, -420.5) projected
  line L541 (257.9886, -420.5) -> (252.2151, -420.5) projected
  line L542 (252.2151, -420.5) -> (249.3284, -415.5) projected
  line L543 (249.3284, -415.5) -> (252.2151, -410.5) projected
  line L544 (252.2151, -410.5) -> (257.9886, -410.5) projected
  line L545 (236.338, -438) -> (239.2247, -433) projected
  line L546 (239.2247, -433) -> (244.9983, -433) projected
  line L547 (244.9983, -433) -> (247.885, -438) projected
  line L548 (247.885, -438) -> (244.9983, -443) projected
  line L549 (244.9983, -443) -> (239.2247, -443) projected
  line L550 (239.2247, -443) -> (236.338, -438) projected
  line L551 (234.8754, -430.5) -> (231.9886, -435.5) projected
  line L552 (231.9886, -435.5) -> (226.2151, -435.5) projected
  line L553 (226.2151, -435.5) -> (223.3284, -430.5) projected
  line L554 (223.3284, -430.5) -> (226.2151, -425.5) projected
  line L555 (226.2151, -425.5) -> (231.9886, -425.5) projected
  line L556 (231.9886, -425.5) -> (234.8754, -430.5) projected
  line L557 (213.2247, -418) -> (218.9983, -418) projected
  line L558 (218.9983, -418) -> (221.885, -423) projected
  line L559 (221.885, -423) -> (218.9983, -428) projected
  line L560 (218.9983, -428) -> (213.2247, -428) projected
  line L561 (213.2247, -428) -> (210.338, -423) projected
  line L562 (210.338, -423) -> (213.2247, -418) projected
  line L563 (205.9886, -440.5) -> (208.8754, -445.5) projected
  line L564 (208.8754, -445.5) -> (205.9886, -450.5) projected
  line L565 (205.9886, -450.5) -> (200.2151, -450.5) projected
  line L566 (200.2151, -450.5) -> (197.3284, -445.5) projected
  line L567 (197.3284, -445.5) -> (200.2151, -440.5) projected
  line L568 (200.2151, -440.5) -> (205.9886, -440.5) projected
  line L569 (187.2247, -413) -> (184.338, -408) projected
  line L570 (184.338, -408) -> (187.2247, -403) projected
  line L571 (187.2247, -403) -> (192.9983, -403) projected
  line L572 (192.9983, -403) -> (195.885, -408) projected
  line L573 (195.885, -408) -> (192.9983, -413) projected
  line L574 (192.9983, -413) -> (187.2247, -413) projected
  line L575 (161.2247, -418) -> (166.9983, -418) projected
  line L576 (166.9983, -418) -> (169.885, -423) projected
  line L577 (169.885, -423) -> (166.9983, -428) projected
  line L578 (166.9983, -428) -> (161.2247, -428) projected
  line L579 (161.2247, -428) -> (158.338, -423) projected
  line L580 (158.338, -423) -> (161.2247, -418) projected
  line L581 (158.338, -438) -> (161.2247, -433) projected
  line L582 (161.2247, -433) -> (166.9983, -433) projected
  line L583 (166.9983, -433) -> (169.885, -438) projected
  line L584 (169.885, -438) -> (166.9983, -443) projected
  line L585 (166.9983, -443) -> (161.2247, -443) projected
  line L586 (161.2247, -443) -> (158.338, -438) projected
  line L587 (132.338, -438) -> (135.2247, -433) projected
  line L588 (135.2247, -433) -> (140.9983, -433) projected
  line L589 (140.9983, -433) -> (143.885, -438) projected
  line L590 (143.885, -438) -> (140.9983, -443) projected
  line L591 (140.9983, -443) -> (135.2247, -443) projected
  line L592 (135.2247, -443) -> (132.338, -438) projected
  line L593 (130.8754, -430.5) -> (127.9886, -435.5) projected
  line L594 (127.9886, -435.5) -> (122.2151, -435.5) projected
  line L595 (122.2151, -435.5) -> (119.3284, -430.5) projected
  line L596 (119.3284, -430.5) -> (122.2151, -425.5) projected
  line L597 (122.2151, -425.5) -> (127.9886, -425.5) projected
  line L598 (127.9886, -425.5) -> (130.8754, -430.5) projected
  line L599 (109.2247, -418) -> (114.9983, -418) projected
  line L600 (114.9983, -418) -> (117.885, -423) projected
  line L601 (117.885, -423) -> (114.9983, -428) projected
  line L602 (114.9983, -428) -> (109.2247, -428) projected
  line L603 (109.2247, -428) -> (106.338, -423) projected
  line L604 (106.338, -423) -> (109.2247, -418) projected
  line L605 (101.9886, -440.5) -> (104.8754, -445.5) projected
  line L606 (104.8754, -445.5) -> (101.9886, -450.5) projected
  line L607 (101.9886, -450.5) -> (96.2151, -450.5) projected
  line L608 (96.2151, -450.5) -> (93.3284, -445.5) projected
  line L609 (93.3284, -445.5) -> (96.2151, -440.5) projected
  line L610 (96.2151, -440.5) -> (101.9886, -440.5) projected
  line L611 (83.2247, -413) -> (80.338, -408) projected
  line L612 (80.338, -408) -> (83.2247, -403) projected
  line L613 (83.2247, -403) -> (88.9983, -403) projected
  line L614 (88.9983, -403) -> (91.885, -408) projected
  line L615 (91.885, -408) -> (88.9983, -413) projected
  line L616 (88.9983, -413) -> (83.2247, -413) projected
  line L617 (57.2247, -448) -> (62.9983, -448) projected
  line L618 (62.9983, -448) -> (65.885, -453) projected
  line L619 (65.885, -453) -> (62.9983, -458) projected
  line L620 (62.9983, -458) -> (57.2247, -458) projected
  line L621 (57.2247, -458) -> (54.338, -453) projected
  line L622 (54.338, -453) -> (57.2247, -448) projected
  line L623 (49.9886, -410.5) -> (52.8754, -415.5) projected
  line L624 (52.8754, -415.5) -> (49.9886, -420.5) projected
  line L625 (49.9886, -420.5) -> (44.2151, -420.5) projected
  line L626 (44.2151, -420.5) -> (41.3284, -415.5) projected
  line L627 (41.3284, -415.5) -> (44.2151, -410.5) projected
  line L628 (44.2151, -410.5) -> (49.9886, -410.5) projected
  line L629 (28.338, -438) -> (31.2247, -433) projected
  line L630 (31.2247, -433) -> (36.9983, -433) projected
  line L631 (36.9983, -433) -> (39.885, -438) projected
  line L632 (39.885, -438) -> (36.9983, -443) projected
  line L633 (36.9983, -443) -> (31.2247, -443) projected
  line L634 (31.2247, -443) -> (28.338, -438) projected
  line L635 (10.9983, -413) -> (5.2247, -413) projected
  line L636 (5.2247, -413) -> (2.338, -408) projected
  line L637 (2.338, -408) -> (5.2247, -403) projected
  line L638 (5.2247, -403) -> (10.9983, -403) projected
  line L639 (10.9983, -403) -> (13.885, -408) projected
  line L640 (13.885, -408) -> (10.9983, -413) projected
  circle A6 centre (268, -105.5) radius 15 projected
  circle A7 centre (180, -105.5) radius 15 projected
  circle A8 centre (92, -105.5) radius 15 projected
  circle A9 centre (76.5, -121) radius 1.75 projected
  circle A10 centre (107.5, -90) radius 1.75 projected
  circle A11 centre (164.5, -121) radius 1.75 projected
  circle A12 centre (195.5, -90) radius 1.75 projected
  circle A13 centre (283.5, -121) radius 1.75 projected
  circle A14 centre (283.5, -90) radius 1.75 projected
  circle A15 centre (252.5, -90) radius 1.75 projected
  circle A16 centre (252.5, -121) radius 1.75 projected
  circle A17 centre (164.5, -90) radius 1.75 projected
  circle A18 centre (195.5, -121) radius 1.75 projected
  circle A19 centre (76.5, -90) radius 1.75 projected
  circle A20 centre (107.5, -121) radius 1.75 projected
  line L641 (375, -480) -> (375, 0) projected
  line L642 (375, 0) -> (-15, 0) projected
  line L643 (-15, 0) -> (-15, -480) projected
  line L644 (-15, -480) -> (375, -480) projected
  circle A21 centre (100, -25) radius 1.75 projected
  circle A22 centre (180, -7.5) radius 1.75 projected
  circle A23 centre (-7.5, -65) radius 1.75 projected
  circle A24 centre (-7.5, -415) radius 1.75 projected
  circle A25 centre (367.5, -65) radius 1.75 projected
  circle A26 centre (367.5, -415) radius 1.75 projected
  circle A27 centre (50, -7.5) radius 1.75 projected
  circle A28 centre (310, -7.5) radius 1.75 projected
  circle A29 centre (310, -472.5) radius 1.75 projected
  circle A30 centre (50, -472.5) radius 1.75 projected
  circle A31 centre (180, -25) radius 1.75 projected
  circle A32 centre (260, -25) radius 1.75 projected
  point P0 (0, 0)
  point P1 (155, -185.5)
  point P2 (205, -185.5)
  dimension "d88" = 50
  dimension "d89" = 25
  dimension "d90" = 80
  constraints: 1 horizontal alignment
  measures "d88" distance of point (155, -185.5) point (205, -185.5)
  measures "d89" horizontal distance of point (205, -185.5) A31.centre
  measures "d90" vertical distance of point (155, -185.5) A7.centre
hole "Hole2" at (155, -185.5, 2) at (205, -185.5, 2) direction (0, 0, -1) diameter 3.2 end through all
sketch "Sketch10" plane through (0, 0, 2) normal (0, 0, 1) x (1, 0, 0)
  circle A0 centre (280, -177.7) radius 4
  circle A1 centre (280, -147.7) radius 4
  circle A2 centre (80, -147.7) radius 4
  circle A3 centre (80, -177.7) radius 4
  point P0 (0, 0)
  constraints: 4 centre point, 8 other
hole "Hole3" at (80, -147.7, 2) at (80, -177.7, 2) at (280, -177.7, 2) at (280, -147.7, 2) direction (0, 0, -1) diameter 3.2 end through all
equation "\"d2\" = d0"
equation "\"d3\" = d2"
equation "\"d4\" = d3"
equation "\"d5\" = d0"
equation "\"d6\" = d0"
equation "\"d25\" = 0.5 * d11"
equation "\"d36\" = d35"
equation "\"d40\" = d39"
equation "\"d41\" = d39"
body "Solid1"
